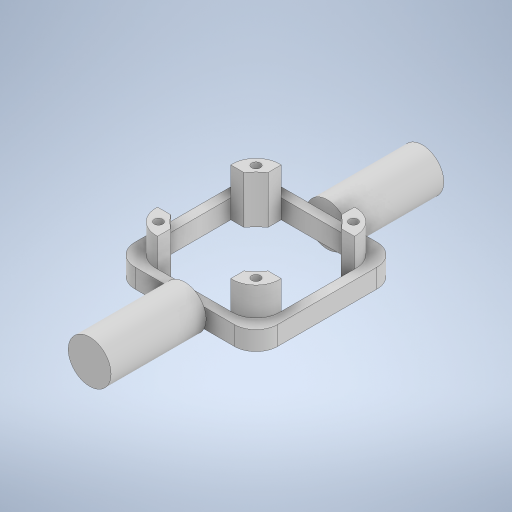
# Autodesk Inventor part: FrontPlateV2
Saved by Autodesk Inventor 2024 (Build 280153000, 153)
## iProperties
Created: 2024-02-08
Part Number: FrontPlateV2
Material: Generic
Document SubType Name: Modeling
Designer: yusuf
Density: 1 g/cm^3
Appearance: Default
Author: yusuf
Autodesk Inventor part; units mm, degrees
ref_plane "YZ Plane" through (0, 0, 0) normal (1, 0, 0) x (0, 1, 0)
ref_plane "XZ Plane" through (0, 0, 0) normal (0, 1, 0) x (-1, 0, 0)
ref_plane "XY Plane" through (0, 0, 0) normal (0, 0, 1) x (1, 0, 0)
sketch "Sketch1" plane through (0, 0, 0) normal (0, 0, 1) x (1, 0, 0)
  circle A0 centre (0, 0) radius 22.5
  dimension "d0" = 45
  constraints: 1 centre point, 1 coincident
  measures "d0" diameter of A0
extrude "Extrusion1" add sketch "Sketch1" along normal blind 100
sketch "Sketch2" plane through (0, 0, 0) normal (0, 0, -1) x (-1, 0, 0)
  circle A0 centre (0, 0) radius 17.5
  point P0 (-6.0869, 16.4073)
  point P1 (4.042, 17.0268)
  dimension "d3" = 35
  constraints: 2 point on circle, 1 centre point, 1 coincident
  measures "d3" diameter of A0
extrude "Extrusion2" cut sketch "Sketch2" against normal blind 90
fillet "Fillet1" radius 0.5 1 edges at (17.5, 0, 0)
fillet "Fillet2" [suppressed]
sketch "Sketch5" plane through (0, 0, 100) normal (0, 0, 1) x (1, 0, 0)
  line L0 (-75, -10) -> (75, -10)
  line L1 (75, -10) -> (75, 10)
  line L2 (75, 10) -> (-75, 10)
  line L3 (-75, 10) -> (-75, -10)
  line L4 (-75, -10) -> (75, 10) construction
  line L5 (75, -10) -> (-75, 10) construction
  point P0 (0, 0)
  dimension "d32" = 150
  dimension "d33" = 20
  constraints: 12 end point, 2 midpoint, 2 parallel, 1 horizontal, 1 perpendicular
  measures "d32" distance of L1.end L2.end
  measures "d33" distance of L0.end L1.end
extrude "Extrusion5" add sketch "Sketch5" along normal blind 150
fillet "Fillet6" radius 22.751 4 edges at (-75, 0, 250) (75, 0, 250) (75, 0, 100) (-75, 0, 100)
sketch "Sketch8" plane through (0, 0, 250) normal (0, 0, 1) x (1, 0, 0)
  circle A0 centre (0, 0) radius 22.5
  dimension "d136" = 45
  constraints: 1 centre point, 1 coincident
  measures "d136" diameter of A0
extrude "Extrusion8" add sketch "Sketch8" along normal blind 100
sketch "Sketch11" plane through (-20.1556, 10, 100) normal (0, 1, 0) x (1, 0, 0)
  line L0 (-44.8444, -140) -> (85.1556, -140)
  line L1 (85.1556, -140) -> (85.1556, -10)
  line L2 (85.1556, -10) -> (-44.8444, -10)
  line L3 (-44.8444, -10) -> (-44.8444, -140)
  line L4 (-44.8444, -140) -> (85.1556, -10) construction
  line L5 (85.1556, -140) -> (-44.8444, -10) construction
  line L6 (-54.8444, -22.751) -> (-54.8444, -127.249) projected
  line L7 (0, -150) -> (40.3113, -150) projected
  line L8 (-54.8444, -127.249) -> (-44.8444, -127.249)
  line L9 (-32.0934, -150) -> (0, -150) projected
  line L10 (-32.0934, -150) -> (-32.0934, -140)
  line L11 (-54.8444, -22.751) -> (-54.8444, -127.249) projected
  line L12 (-54.8444, -22.751) -> (-44.8444, -22.751)
  arc A0 (-32.0934, 0) -> (-54.8444, -22.751) centre (-32.0934, -22.751) ccw projected
  line L13 (-32.0934, 0) -> (-32.0934, -10)
  line L14 (72.4046, 0) -> (40.3113, 0) projected
  line L15 (72.4046, 0) -> (72.4046, -10)
  arc A1 (95.1556, -22.751) -> (72.4046, 0) centre (72.4046, -22.751) ccw projected
  line L16 (95.1556, -22.751) -> (85.1556, -22.751)
  line L17 (40.3113, -150) -> (72.4046, -150) projected
  line L18 (72.4046, -150) -> (72.4046, -140)
  line L19 (95.1556, -22.751) -> (95.1556, -127.249) projected
  line L20 (95.1556, -127.249) -> (85.1556, -127.249)
  line L21 (-44.8444, -75) -> (-44.8444, -36.5)
  line L22 (-44.8444, -75) -> (-44.8444, -113.5)
  line L23 (-44.8444, -36.5) -> (-31.0444, -36.5)
  line L24 (20.1556, -10) -> (-18.3444, -10)
  line L25 (20.1556, -10) -> (58.6556, -10)
  line L26 (-18.3444, -10) -> (-18.3444, -23.8)
  arc A2 (-18.3444, -23.8) -> (-31.0444, -36.5) centre (20.327, -75.1714) ccw
  line L27 (20.1556, -140) -> (-18.3444, -140)
  line L28 (20.1556, -140) -> (58.6556, -140)
  line L29 (85.1556, -75) -> (85.1556, -113.5)
  line L30 (85.1556, -75) -> (85.1556, -36.5)
  line L31 (20.1556, -10) -> (58.6556, -10)
  line L32 (-44.8444, -113.5) -> (-31.0444, -113.5)
  line L33 (-18.3444, -140) -> (-18.3444, -126.2)
  line L34 (58.6556, -140) -> (58.6556, -126.2)
  line L35 (85.1556, -113.5) -> (71.3556, -113.5)
  line L36 (85.1556, -36.5) -> (71.3556, -36.5)
  line L37 (58.6556, -10) -> (58.6556, -23.8)
  arc A3 (58.6556, -126.2) -> (71.3556, -113.5) centre (19.9843, -74.8286) ccw
  arc A4 (-31.0444, -113.5) -> (-18.3444, -126.2) centre (20.327, -74.8286) ccw
  arc A5 (71.3556, -36.5) -> (58.6556, -23.8) centre (19.9843, -75.1714) ccw
  point P0 (20.1556, 100)
  point P1 (20.1556, -75)
  dimension "d72" = 130
  dimension "d73" = 130
  dimension "d74" = 75
  dimension "d75" = 75
  dimension "d84" = 38.5
  dimension "d85" = 38.5
  dimension "d86" = 13.8
  dimension "d87" = 38.5
  dimension "d88" = 38.5
  dimension "d89" = 13.8
  dimension "d90" = 64.3
  dimension "d96" = 38.5
  dimension "d97" = 38.5
  dimension "d98" = 38.5
  dimension "d99" = 38.5
  dimension "d100" = 13.8
  dimension "d101" = 13.8
  dimension "d102" = 13.8
  dimension "d103" = 13.8
  dimension "d104" = 13.8
  dimension "d105" = 13.8
  dimension "d106" = 64.3
  dimension "d107" = 64.3
  dimension "d108" = 64.3
  constraints: 62 end point, 20 point on line, 8 point on circle, 6 midpoint, 5 horizontal, 5 perpendicular, 4 centre point, 4 vertical, 3 equal length
  measures "d72" distance of L1.end L2.end
  measures "d73" distance of L0.end L1.end
  measures "d74" distance from line of point (20.156, -75) L6
  measures "d75" distance from line of L7 point (20.156, -75)
  measures "d84" distance of L21.start L21.end
  measures "d85" distance of L21.start L22.end
  measures "d86" distance of L21.end L23.end
  measures "d87" distance of L24.start L24.end
  measures "d88" distance of L24.start L25.end
  measures "d89" distance of L24.end L26.end
  measures "d90" radius of A2
  measures "d96" distance of L27.start L27.end
  measures "d97" distance of L27.start L28.end
  measures "d98" distance of L29.start L29.end
  measures "d99" distance of L29.start L30.end
  measures "d100" distance of L22.end L32.end
  measures "d101" distance of L27.end L33.end
  measures "d102" distance of L28.end L34.end
  measures "d103" distance of L29.end L35.end
  measures "d104" distance of L30.end L36.end
  measures "d105" distance of L25.end L37.end
  measures "d106" radius of A3
  measures "d107" radius of A4
  measures "d108" radius of A5
extrude "Extrusion10" cut sketch "Sketch11" against normal blind 20 contours L33 A4 L32 L3 L23 A2 L26 L2 L37 A5 L36 L1 L35 A3 L34 L0
sketch "Sketch12" plane through (-20.1556, 10, 100) normal (0, 1, 0) x (1, 0, 0)
  circle A0 centre (-31.1094, -23.735) radius 4.5
  line L0 (-44.8444, -36.5) -> (-31.0444, -36.5) projected
  line L1 (-44.8444, -113.5) -> (-44.8444, -36.5) projected
  circle A1 centre (-31.1094, -126.265) radius 4.5
  circle A2 centre (71.4206, -126.265) radius 4.5
  circle A3 centre (71.4206, -23.735) radius 4.5
  line L2 (-31.0444, -113.5) -> (-44.8444, -113.5) projected
  line L3 (85.1556, -113.5) -> (71.3556, -113.5) projected
  line L4 (85.1556, -36.5) -> (85.1556, -113.5) projected
  line L5 (71.3556, -36.5) -> (85.1556, -36.5) projected
  point P0 (20.1556, 100)
  point P1 (-28.3394, -127.249)
  dimension "d91" = 9
  dimension "d92" = 12.765
  dimension "d93" = 13.735
  dimension "d109" = 9
  dimension "d110" = 9
  dimension "d111" = 9
  dimension "d112" = 12.765
  dimension "d113" = 13.735
  dimension "d114" = 12.765
  dimension "d115" = 13.735
  dimension "d116" = 13.735
  dimension "d117" = 12.765
  constraints: 4 centre point, 1 other
  measures "d91" diameter of A0
  measures "d92" distance from line of A0.centre L0
  measures "d109" diameter of A1
  measures "d110" diameter of A2
  measures "d111" diameter of A3
  measures "d112" distance from line of L2 A1.centre
  measures "d114" distance from line of L3 A2.centre
  measures "d115" distance from line of L4 A2.centre
  measures "d116" distance from line of L4 A3.centre
  measures "d117" distance from line of L5 A3.centre
extrude "Extrusion11" cut sketch "Sketch12" along normal mid plane 50
sketch "Sketch13" plane through (-20.1556, 10, 100) normal (0, 1, 0) x (1, 0, 0)
  line L0 (-44.8444, -113.5) -> (-44.8444, -36.5) projected
  line L1 (58.6556, -140) -> (-18.3444, -140) projected
  arc A0 (-44.8444, -113.5) -> (-18.3444, -140) centre (-19.8923, -115.048) ccw
  line L2 (-18.3444, -10) -> (-18.3444, -23.8) projected
  arc A1 (-18.3444, -10) -> (-44.8444, -36.5) centre (-19.8923, -34.952) ccw
  line L3 (85.1556, -113.5) -> (85.1556, -36.5) projected
  arc A2 (58.6556, -140) -> (85.1556, -113.5) centre (60.2036, -115.048) ccw
  line L4 (85.1556, -36.5) -> (71.3556, -36.5) projected
  line L5 (58.6556, -23.8) -> (58.6556, -10) projected
  arc A3 (85.1556, -36.5) -> (58.6556, -10) centre (60.2036, -34.952) ccw
  line L6 (-18.3444, -126.2) -> (-18.3444, -140) projected
  line L7 (-18.3444, -140) -> (-18.3444, -126.2)
  arc A4 (-31.0444, -113.5) -> (-18.3444, -126.2) centre (20.327, -74.8286) ccw projected
  line L8 (-44.8444, -113.5) -> (-31.0444, -113.5)
  arc A5 (-31.0444, -113.5) -> (-18.3444, -126.2) centre (20.327, -74.8286) ccw
  line L9 (-31.0444, -36.5) -> (-44.8444, -36.5) projected
  line L10 (-44.8444, -36.5) -> (-31.0444, -36.5)
  line L11 (-18.3444, -10) -> (-18.3444, -23.8)
  line L12 (58.6556, -10) -> (58.6556, -23.8)
  line L13 (71.3556, -36.5) -> (85.1556, -36.5)
  line L14 (85.1556, -113.5) -> (71.3556, -113.5) projected
  line L15 (71.3556, -113.5) -> (85.1556, -113.5)
  arc A6 (-18.3444, -23.8) -> (-31.0444, -36.5) centre (20.327, -75.1714) ccw projected
  arc A7 (-18.3444, -23.8) -> (-31.0444, -36.5) centre (20.327, -75.1714) ccw
  arc A8 (71.3556, -36.5) -> (58.6556, -23.8) centre (19.9843, -75.1714) ccw
  line L16 (58.6556, -140) -> (58.6556, -126.2) projected
  line L17 (58.6556, -140) -> (58.6556, -126.2)
  arc A9 (58.6556, -126.2) -> (71.3556, -113.5) centre (19.9843, -74.8286) ccw projected
  arc A10 (58.6556, -126.2) -> (71.3556, -113.5) centre (19.9843, -74.8286) ccw
  point P0 (20.1556, 100)
  dimension "d118" = 25
  dimension "d119" = 25
  dimension "d120" = 25
  dimension "d121" = 25
  dimension "d122" = 64.3
  dimension "d125" = 64.3
  dimension "d126" = 64.3
  dimension "d127" = 64.3
  constraints: 16 end point, 16 point on circle, 8 centre point, 5 collinear, 1 horizontal, 1 perpendicular, 1 vertical
  measures "d118" radius of A0
  measures "d119" radius of A1
  measures "d120" radius of A2
  measures "d121" radius of A3
  measures "d122" radius of A5
  measures "d125" radius of A7
  measures "d126" radius of A8
  measures "d127" radius of A10
extrude "Extrusion12" add sketch "Sketch13" along normal blind 30
sketch "Sketch14" plane through (-20.1556, -10, 100) normal (0, -1, 0) x (1, 0, 0)
  circle A0 centre (-31.1094, 23.735) radius 4.5 projected
  circle A1 centre (-31.1094, 23.735) radius 4.5
  circle A2 centre (-31.1094, 126.265) radius 4.5 projected
  circle A3 centre (-31.1094, 126.265) radius 4.5
  circle A4 centre (71.4206, 126.265) radius 4.5 projected
  circle A5 centre (71.4206, 126.265) radius 4.5
  circle A6 centre (71.4206, 23.735) radius 4.5 projected
  circle A7 centre (71.4206, 23.735) radius 4.5
  point P0 (20.1556, -100)
  dimension "d130" = 9
  dimension "d131" = 9
  dimension "d132" = 9
  dimension "d133" = 9
  constraints: 4 centre point, 4 coincident
  measures "d130" diameter of A1
  measures "d131" diameter of A5
  measures "d132" diameter of A7
  measures "d133" diameter of A3
extrude "Extrusion13" cut sketch "Sketch14" against normal blind 100
equation "\"d112\" = d92"
equation "\"d113\" = d93"
equation "\"d114\" = d112"
equation "\"d115\" = d113"
equation "\"d116\" = d115"
equation "\"d117\" = d114"
body "Solid1"
